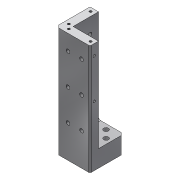
# Autodesk Inventor part: BC-10016
Saved by Autodesk Inventor 2016 (Build 200138000, 138)
## iProperties
Created: 2015-11-09
Part Number: BC-10016
Project: DIPOLO BC-3T- SIRIUS
Cost Center: 1504002005
Material: Alumínio 7075
Document SubType Name: Modeling
Designer: reinaldo.basilio
Density: 2.81 g/cm^3
Appearance: Aluminum - Polished
Mass: 982.39 g
Surface Area: 599.676 cm^2
Volume: 349.605 cm^3
Description: Fixador frontal dos blocos magnéticos.
RuleStatus: InUse
AfterMaterialChange0: file://_iMaterial
AfterAnyiPropertyChange0: file://_iMaterial
AfterDocNew0: file://_Naming_par
AfterDocNew1: file://_NameStart
AfterDocNew2: file://_NameStart1
AfterDocNew3: file://_Materiais
DocNumber: XXXXX-XXX-XXXX-00-001.ipt
Folder: .
Title: DIPOLO BC-3T- SIRIUS
Author: reinaldo.basilio
Autodesk Inventor part; units mm, degrees
ref_plane "YZ Plane" through (0, 0, 0) normal (1, 0, 0) x (0, 1, 0)
ref_plane "XZ Plane" through (0, 0, 0) normal (0, 1, 0) x (-1, 0, 0)
ref_plane "XY Plane" through (0, 0, 0) normal (0, 0, 1) x (1, 0, 0)
sketch "Sketch5" plane through (0, 0, 0) normal (0, 0, 1) x (1, 0, 0)
  line L0 (-30, 30) -> (30, 30)
  line L1 (30, 30) -> (30, -30)
  line L2 (30, -30) -> (-30, -30)
  line L3 (-30, -30) -> (-30, 30)
  point P0 (0, 0)
  point P1 (0, 30)
  point P2 (30, 0)
  dimension "d8" = 60
  dimension "d9" = 60
  constraints: 8 end point, 2 midpoint, 2 parallel, 1 horizontal, 1 horizontal alignment, 1 perpendicular, 1 vertical alignment
  measures "d8" distance of L0.start L0.end
  measures "d9" distance of L2.end L0.start
extrude "Extrusion5" add sketch "Sketch5" along normal blind 195
sketch "Sketch8" plane through (0, 0, 195) normal (0, 0, 1) x (1, 0, 0)
  line L0 (-30, -30) -> (30, -30) projected
  line L1 (30, -30) -> (30, 30) projected
  line L2 (-30, 30) -> (15, 30)
  line L3 (15, 30) -> (15, -15)
  line L4 (15, -15) -> (-30, -15)
  line L5 (-30, -15) -> (-30, 30)
  point P0 (0, 0)
  dimension "d25" = 15
  dimension "d26" = 15
  constraints: 8 end point, 2 parallel, 1 horizontal, 1 perpendicular
  measures "d25" distance between parallel lines of L4 L0
  measures "d26" distance between parallel lines of L1 L3
extrude "Extrusion8" cut sketch "Sketch8" against normal blind 165
sketch "Sketch9" plane through (0, 0, 30) normal (0, 0, 1) x (1, 0, 0)
  circle A0 centre (6, 7.5) radius 4
  circle A1 centre (-21, 7.5) radius 4
  line L0 (30, -30) -> (30, 30) projected
  line L1 (-30, -30) -> (30, -30) projected
  circle A2 centre (6, 7.5) radius 8
  line L2 (-30, -15) -> (-30, 30) projected
  line L3 (15, 30) -> (15, -15) projected
  circle A3 centre (-7.5, -6) radius 4
  circle A4 centre (-7.5, 21) radius 4
  line L4 (15, -15) -> (-30, -15) projected
  point P0 (0, 0)
  point P1 (15, 7.5)
  point P2 (-30, 7.5)
  point P3 (-7.5, -15)
  dimension "d29" = 24
  dimension "d31" = 8
  dimension "d32" = 16
  dimension "d41" = 9
  dimension "d42" = 27
  dimension "d43" = 27
  dimension "d44" = 13.5
  dimension "d45" = 9
  constraints: 5 centre point, 3 equal radius, 3 midpoint, 2 horizontal alignment, 2 vertical alignment, 1 coincident
  measures "d29" distance from line of A0.centre L0
  measures "d31" diameter of A0
  measures "d32" diameter of A2
  measures "d41" distance from line of L2 A1.centre
  measures "d42" distance of A1.centre A2.centre
  measures "d43" distance of A3.centre A4.centre
  measures "d44" horizontal distance of A3.centre A1.centre
  measures "d45" distance from line of L3 A0.centre
hole "Hole1" at (6, 7.5, 30) at (-21, 7.5, 30) at (-7.5, 21, 30) at (-7.5, -6, 30) direction (0, 0, -1) diameter 8.5 end through all
fillet "Fillet2" radius 4 1 edges at (-7.5, -15, 30)
sketch "Sketch10" plane through (15, -15, 195) normal (-1, 0, 0) x (0, 0, 1)
  line L0 (-165, 45) -> (0, 45) projected
  circle A0 centre (-27.5, 30) radius 4
  circle A1 centre (-27.5, 6) radius 4
  circle A2 centre (-82.5, 30) radius 4
  circle A3 centre (-82.5, 6) radius 4
  circle A4 centre (-137.5, 30) radius 4
  circle A5 centre (-137.5, 6) radius 4
  line L1 (-195, -15) -> (0, -15) projected
  line L2 (0, 45) -> (0, 0) projected
  line L3 (-165, 45) -> (-165, 4) projected
  point P0 (-195, 15)
  dimension "d47" = 15
  dimension "d48" = 21
  dimension "d49" = 8
  dimension "d57" = 27.5
  dimension "d58" = 55
  dimension "d59" = 55
  dimension "d60" = 27.5
  constraints: 6 centre point, 5 equal radius, 4 horizontal alignment, 3 vertical alignment
  measures "d47" distance from line of A0.centre L0
  measures "d48" distance from line of A1.centre L1
  measures "d49" diameter of A1
  measures "d57" distance from line of A0.centre L2
  measures "d58" distance of A2.centre A0.centre
  measures "d59" distance of A4.centre A2.centre
  measures "d60" distance from line of A4.centre L3
hole "Hole2" at (15, 15, 167.5) at (15, -9, 167.5) at (15, 15, 112.5) at (15, -9, 112.5) at (15, -9, 57.5) at (15, 15, 57.5) direction (1, 0, 0) diameter 6.647 end through all thread size "M8x1.25" class "6H" standard "ISO Metric profile"
sketch "Sketch11" plane through (-30, -15, 195) normal (0, 1, 0) x (1, 0, 0)
  line L0 (45, 0) -> (0, 0) projected
  circle A0 centre (15, 137.5) radius 4
  circle A1 centre (39, 137.5) radius 4
  circle A2 centre (15, 82.5) radius 4
  circle A3 centre (39, 82.5) radius 4
  circle A4 centre (15, 27.5) radius 4
  circle A5 centre (39, 27.5) radius 4
  line L1 (60, 195) -> (60, 0) projected
  point P0 (30, 195)
  dimension "d63" = 8
  dimension "d65" = 55
  dimension "d66" = 55
  dimension "d68" = 24
  dimension "d69" = 21
  dimension "d70" = 27.5
  constraints: 6 centre point, 5 equal radius, 4 vertical alignment, 3 horizontal alignment
  measures "d63" diameter of A1
  measures "d65" distance of A2.centre A0.centre
  measures "d66" distance of A4.centre A2.centre
  measures "d68" distance of A4.centre A5.centre
  measures "d69" distance from line of L1 A5.centre
  measures "d70" distance from line of L0 A4.centre
hole "Hole3" at (9, -15, 167.5) at (-15, -15, 167.5) at (9, -15, 112.5) at (-15, -15, 112.5) at (9, -15, 57.5) at (-15, -15, 57.5) direction (0, -1, 0) diameter 6.647 end through all thread size "M8x1.25" class "6H" standard "ISO Metric profile"
sketch "Sketch12" plane through (-30, -30, 0) normal (-1, 0, 0) x (0, 0, 1)
  line L0 (195, 15) -> (195, 0) projected
  circle A0 centre (176.25, 7.5) radius 3
  circle A1 centre (106.25, 7.5) radius 3
  point P0 (0, 30)
  point P1 (195, 7.5)
  dimension "d78" = 70
  dimension "d79" = 18.75
  dimension "d80" = 6
  constraints: 2 centre point, 2 horizontal alignment, 1 equal radius, 1 midpoint
  measures "d78" distance of A1.centre A0.centre
  measures "d79" distance from line of L0 A0.centre
  measures "d80" diameter of A0
hole "Hole4" at (-30, -22.5, 176.25) at (-30, -22.5, 106.25) direction (1, 0, 0) diameter 4.134 depth 15 tip angle 118 thread size "M5x0.8" class "6H" standard "ISO Metric profile"
sketch "Sketch13" plane through (-30, 30, 0) normal (0, 1, 0) x (1, 0, 0)
  line L0 (60, -195) -> (45, -195) projected
  circle A0 centre (52.5, -176.25) radius 3
  circle A1 centre (52.5, -106.25) radius 3
  point P0 (30, 0)
  point P1 (52.5, -195)
  dimension "d88" = 18.75
  dimension "d89" = 70
  dimension "d90" = 6
  constraints: 2 centre point, 2 vertical alignment, 1 equal radius, 1 midpoint
  measures "d88" distance of A0.centre point (52.5, -195)
  measures "d89" distance of A0.centre A1.centre
  measures "d90" diameter of A0
hole "Hole5" at (22.5, 30, 176.25) at (22.5, 30, 106.25) direction (0, -1, 0) diameter 4.134 depth 15 tip angle 118 thread size "M5x0.8" class "6H" standard "ISO Metric profile"
chamfer "Chamfer1" distance 5 angle 45 2 edges at (30, -30, 97.5) (-30, 30, 15)
chamfer "Chamfer2" distance 2 angle 45 2 edges at (30, 30, 97.5) (-30, -30, 97.5)
sketch "Sketch14" plane through (0, 0, 195) normal (0, 0, 1) x (1, 0, 0)
  line L0 (-28, -30) -> (25, -30) projected
  line L1 (30, -25) -> (30, 28) projected
  line L2 (15, -15) -> (-30, -15) projected
  circle A0 centre (15, -22.5) radius 2.5
  circle A1 centre (-23.5, -22.5) radius 2.5
  circle A2 centre (22.5, 23.5) radius 2.5
  line L3 (28, 30) -> (15, 30) projected
  line L4 (-30, -15) -> (-30, -28) projected
  circle A3 centre (22.5, -15) radius 2.5
  point P0 (0, 0)
  dimension "d104" = 15
  dimension "d105" = 7.5
  dimension "d106" = 5
  dimension "d107" = 7.5
  dimension "d116" = 6.5
  dimension "d117" = 6.5
  dimension "d119" = 45
  dimension "d120" = 45
  constraints: 4 centre point, 3 equal radius, 1 horizontal alignment, 1 vertical alignment
  measures "d104" distance between parallel lines of L2 L0
  measures "d105" distance from line of L0 A1.centre
  measures "d106" diameter of A0
  measures "d107" distance from line of L1 A2.centre
  measures "d116" distance from line of L4 A1.centre
  measures "d117" distance from line of L3 A2.centre
  measures "d119" distance from line of A0.centre L4
  measures "d120" distance from line of A3.centre L3
hole "Hole6" at (-23.5, -22.5, 195) at (15, -22.5, 195) at (22.5, 23.5, 195) at (22.5, -15, 195) direction (0, 0, -1) diameter 4.134 depth 15 tip angle 118 thread size "M5x0.8" class "6H" standard "ANSI Metric M Profile"
equation "\"d26\" = d25"
equation "\"d44\" = 0.5 * d43"
equation "\"d107\" = d105"
equation "\"d117\" = d116"
equation "\"d120\" = d119"
body "Solid5"
